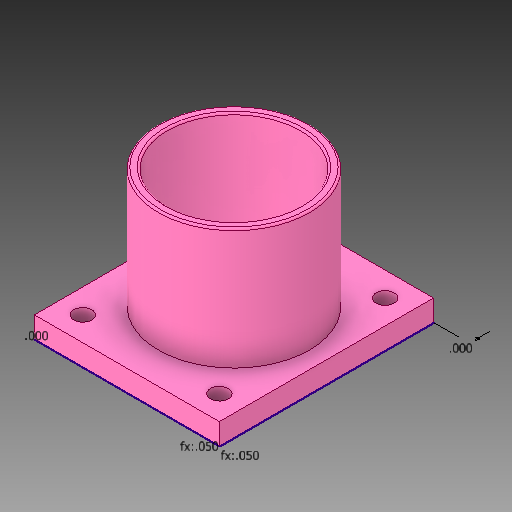
# Autodesk Inventor part: TelescopeAttachementForCase
Saved by Autodesk Inventor 2019.3 (Build 233278000, 278)
## iProperties
Created: 2018-12-18
Part Number: TelescopeAttachementForCase
Material: Polypropylene
Document SubType Name: Modeling
Designer: steele
Density: 0.899 g/cm^3
Appearance: Pink
Author: steele
Autodesk Inventor part; units mm, degrees
ref_plane "YZ Plane" through (0, 0, 0) normal (1, 0, 0) x (0, 1, 0)
ref_plane "XZ Plane" through (0, 0, 0) normal (0, 1, 0) x (-1, 0, 0)
ref_plane "XY Plane" through (0, 0, 0) normal (0, 0, 1) x (1, 0, 0)
sketch "Sketch1" plane through (0, 0, 0) normal (0, 1, 0) x (-1, 0, 0)
  line L0 (19.431, 22.5) -> (-19.431, 22.5)
  line L1 (-19.431, 22.5) -> (-19.431, -22.5)
  line L2 (-19.431, -22.5) -> (19.431, -22.5)
  line L3 (19.431, -22.5) -> (19.431, 22.5)
  line L4 (19.431, 22.5) -> (-19.431, -22.5) construction
  line L5 (-19.431, 22.5) -> (19.431, -22.5) construction
  point P0 (0, 0)
  dimension "d0" = 38.862
  dimension "d1" = 45
  constraints: 12 end point, 2 midpoint, 2 parallel, 1 horizontal, 1 perpendicular
  measures "d0" distance of L0.start L0.end
  measures "d1" distance of L2.end L0.start
extrude "ExtrusionForFloor" add sketch "Sketch1" against normal blind 4.445
sketch "Sketch4" plane through (0, 0, 0) normal (0, 1, 0) x (1, 0, 0)
  line L0 (-5, -5) -> (5, -5)
  line L1 (5, -5) -> (5, 5)
  line L2 (5, 5) -> (-5, 5)
  line L3 (-5, 5) -> (-5, -5)
  line L4 (-5, -5) -> (5, 5) construction
  line L5 (5, -5) -> (-5, 5) construction
  point P0 (0, 0)
  dimension "d21" = 10
  constraints: 12 end point, 2 midpoint, 2 parallel, 2 perpendicular, 1 horizontal
  measures "d21" distance of L0.start L0.end
extrude "ExtrusionForCameraHole" cut sketch "Sketch4" against normal through all
sketch "Sketch5" plane through (0, -4.445, 0) normal (0, -1, 0) x (1, 0, 0)
  line L0 (18.161, 21.23) -> (-18.161, 21.23)
  line L1 (-18.161, 21.23) -> (-18.161, -21.23)
  line L2 (-18.161, -21.23) -> (18.161, -21.23)
  line L3 (18.161, -21.23) -> (18.161, 21.23)
  line L4 (18.161, 21.23) -> (-18.161, -21.23) construction
  line L5 (-18.161, 21.23) -> (18.161, -21.23) construction
  line L6 (19.431, -22.5) -> (19.431, 22.5) projected
  line L7 (19.431, 22.5) -> (-19.431, 22.5) projected
  line L8 (19.431, 22.5) -> (-19.431, 22.5)
  line L9 (-19.431, 22.5) -> (-19.431, -22.5)
  line L10 (-19.431, -22.5) -> (19.431, -22.5)
  line L11 (19.431, -22.5) -> (19.431, 22.5)
  line L12 (-19.431, 22.5) -> (-19.431, -22.5) projected
  line L13 (-19.431, -22.5) -> (19.431, -22.5) projected
  point P0 (0, 0)
  dimension "d24" = 1.27
  dimension "d25" = 1.27
  dimension "d41" = 0
  dimension "d43" = 0
  constraints: 20 end point, 4 parallel, 2 horizontal, 2 midpoint, 2 perpendicular
  measures "d24" distance between parallel lines of L3 L6
  measures "d25" distance between parallel lines of L7 L0
  measures "d41" distance between parallel lines of L9 L12
  measures "d43" distance between parallel lines of L13 L10
sketch "Sketch7" plane through (0, 0, 0) normal (0, 1, 0) x (1, 0, 0)
  circle A0 centre (0, 0) radius 15.875
  circle A1 centre (0, 0) radius 13.97
  dimension "d32" = 31.75
  dimension "d33" = 27.94
  constraints: 2 centre point, 2 coincident
  measures "d32" diameter of A0
  measures "d33" diameter of A1
extrude "ExtrusionForEyepieceAttachement" add sketch "Sketch7" along normal blind 25.4
sketch "Sketch19" plane through (0, 0, 0) normal (0, 1, 0) x (1, 0, 0)
  circle A0 centre (-14.351, 17.42) radius 1.2192 projected
  circle A1 centre (-14.351, -17.42) radius 1.2192 projected
  circle A2 centre (14.351, -17.42) radius 1.2192 projected
  circle A3 centre (14.351, 17.42) radius 1.2192 projected
  line L0 (19.431, -22.5) -> (19.431, 22.5) projected
  line L1 (-19.431, 22.5) -> (-19.431, -22.5) projected
  line L2 (-19.431, -22.5) -> (19.431, -22.5) projected
  line L3 (19.431, 22.5) -> (-19.431, 22.5) projected
  point P0 (0, 0)
  dimension "d104" = 5.08
  dimension "d105" = 5.08
  dimension "d106" = 5.08
  dimension "d107" = 5.08
  dimension "d108" = 5.08
  dimension "d109" = 5.08
  dimension "d110" = 5.08
  dimension "d111" = 5.08
  constraints: 4 coincident
  measures "d104" distance from line of A2.centre L0
  measures "d105" distance from line of A1.centre L1
  measures "d106" distance from line of A1.centre L2
  measures "d107" distance from line of point (-14.351, 17.42) L3
  measures "d108" distance from line of A0.centre L1
  measures "d109" distance from line of A3.centre L0
  measures "d110" distance from line of L2 A2.centre
  measures "d111" distance from line of A3.centre L3
hole "Hole5" at (-14.351, 0, -17.42) at (-14.351, 0, 17.42) at (14.351, 0, 17.42) at (14.351, 0, -17.42) direction (0, -1, 0) diameter 3.81 end through all clearance for "Flat Head Machine Screw (82)" size "#6" standard "Ansi Unified Screw Threads"
fillet "Fillet3" radius 0.3969 2 edges at (-15.875, 25.4, 0) (-13.97, 25.4, 0)
fillet "Fillet4" radius 1 4 edges at (-5, -4.445, 0) (0, -4.445, -5) (5, -4.445, 0) (0, -4.445, 5)
fillet "Fillet5" radius 1 4 edges at (0, 0, 5) (-5, 0, 0) (0, 0, -5) (5, 0, 0)
chamfer "Chamfer2" distance 3.175 angle 45 1 edges at (-13.97, 0, 0)
equation "\"d1\" = CaseWidth"
equation "\"d21\" = PiCameraLensCover"
equation "\"d24\" = CaseWallThickness"
equation "\"d25\" = CaseWallThickness"
equation "\"d32\" = EyepieceOutsideDiameter"
equation "\"d33\" = EyepieceInnerDiameter"
equation "\"d34\" = EyepieceAdapterLength"
equation "\"PiCameraLength\" = 23.862"
equation "\"PiCameraWidth\" = 25"
equation "\"PiCameraLensCover\" = 10"
equation "\"EyepieceAdapterLength\" = 25.4"
equation "\"OffsetForBoltPattern\" = 3.175"
equation "\"FloorThickness\" = 1.905"
equation "\"SlotForEyepiece\" = 2.54"
equation "\"CaseWidth\" = 45"
equation "\"CaseWallThickness\" = 1.27"
equation "\"EyepieceOutsideDiameter\" = 31.75"
equation "\"EyepieceInnerDiameter\" = 27.94"
body "Solid1"
